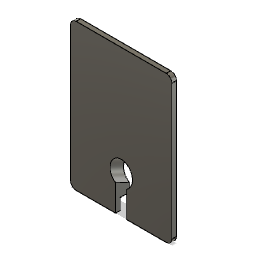
JRCNC0008 v3 (Autodesk Fusion 360 design; units mm, degrees)
Autodesk Fusion 360 part; units mm, degrees
sketch "Sketch1" plane through (0, 0, 0) normal (0, 0, 1) x (1, 0, 0)
  line L0 (0, 0) -> (114.3, 0)
  line L1 (114.3, 0) -> (114.3, 165.1)
  line L2 (114.3, 165.1) -> (0, 165.1)
  line L3 (0, 165.1) -> (0, 0)
  dimension "d19" = 114.3
  dimension "d20" = 165.1
  constraint horizontal L0
  constraint vertical L1
  constraint horizontal L2
  constraint vertical L3
  constraint coincident L0.start L3.end
  measures "d19" distance of L0.start L0.end
  measures "d20" distance of L0.start L2.end
extrude "Extrude1" add sketch "Sketch1" along normal blind 15.24
ref_plane "WorkPlane2" through (57.15, 165.1, 15.24) normal (0, 0.422618, 0.906308) x (-1, 0, 0)
sketch "Sketch2" plane through (57.15, 161.2085, 17.0546) normal (0, 0.422618, 0.906308) x (-1, 0, 0)
  circle A0 centre (0, 107.4662) radius 12.7
  line L0 (-57.15, -4.2938) -> (57.15, -4.2938) construction
  line L1 (0, -4.2938) -> (0, 107.4662)
  point P0 (57.15, -4.2938)
  point P1 (-57.15, -4.2938)
  dimension "d21" = 111.76
  dimension "d23" = 25.4
  constraint horizontal L0
  constraint coincident P0 L0.end
  constraint coincident P1 L0.start
  constraint midpoint L0 L1.start
  constraint perpendicular L0 L1
  constraint coincident A0.centre L1.end
  measures "d21" distance of L1.start A0.centre
  measures "d23" diameter of A0
extrude "Extrude2" cut sketch "Sketch2" against normal blind 203.2
sketch "Sketch3" plane through (114.3, 0, 0) normal (1, 0, 0) x (0, 1, 0)
  line L0 (0, 0) -> (165.1, 0)
  line L1 (165.1, 0) -> (165.1, 15.24)
  line L2 (165.1, 15.24) -> (0, 15.24)
  line L3 (0, 15.24) -> (0, 0)
  line L4 (133.35, 15.24) -> (88.9, 15.24)
  line L5 (88.9, 15.24) -> (88.9, 80.645)
  line L6 (88.9, 80.645) -> (133.35, 80.645)
  line L7 (133.35, 80.645) -> (133.35, 15.24)
  line L8 (133.35, 72.39) -> (107.95, 72.39)
  line L9 (107.95, 72.39) -> (107.95, 43.815)
  line L10 (107.95, 43.815) -> (133.35, 43.815)
  line L11 (133.35, 43.815) -> (133.35, 72.39)
  dimension "d22" = 28.575
  dimension "d24" = 57.15
  dimension "d25" = 25.4
  dimension "d26" = 8.255
  dimension "d27" = 19.05
  dimension "d28" = 88.9
  constraint horizontal L4
  constraint vertical L5
  constraint horizontal L6
  constraint vertical L7
  constraint coincident L2 L4.start
  constraint horizontal L8
  constraint vertical L9
  constraint horizontal L10
  constraint vertical L11
  constraint coincident L7 L8.start
  measures "d22" distance of L8.end L9.end
  measures "d24" distance of L4 L8
  measures "d25" distance of L8.start L8.end
  measures "d26" distance of L6.end L8
  measures "d27" distance of L5 L9
  measures "d28" distance of L3 L5
sketch "Sketch4" plane through (0, 0, 0) normal (0, 0, -1) x (1, 0, 0)
  line L0 (0, 0) -> (0, -165.1)
  line L1 (0, -165.1) -> (114.3, -165.1)
  line L2 (114.3, -165.1) -> (114.3, 0)
  line L3 (114.3, 0) -> (0, 0)
  line L4 (0, 0) -> (114.3, 0)
  line L5 (114.3, 0) -> (114.3, -165.1)
  line L6 (114.3, -165.1) -> (0, -165.1)
  line L7 (0, -165.1) -> (0, 0)
  line L8 (57.15, 0) -> (57.15, -165.1) construction
  line L9 (101.6, -12.7) -> (12.7, -12.7)
  line L10 (12.7, -12.7) -> (12.7, -152.4)
  line L11 (12.7, -152.4) -> (101.6, -152.4)
  line L12 (101.6, -152.4) -> (101.6, -12.7)
  line L13 (101.6, -12.7) -> (12.7, -152.4) construction
  line L14 (12.7, -12.7) -> (101.6, -152.4) construction
  line L15 (0, -82.55) -> (114.3, -82.55) construction
  ellipse E0 centre (57.15, -34.68) end of major axis (57.15, -48.6929) minor radius 12.7
  point P0 (57.15, -82.55)
  dimension "d17" = 88.9
  dimension "d18" = 139.7
  constraint horizontal L4
  constraint vertical L5
  constraint horizontal L6
  constraint vertical L7
  constraint coincident L1.end L2.start
  constraint coincident L0.start L3.end
  constraint midpoint L4 L8.start
  constraint midpoint L6 L8.end
  constraint horizontal L9
  constraint perpendicular L9 L10
  constraint parallel L9 L11
  constraint parallel L10 L12
  constraint coincident L13 P0
  constraint coincident L14 P0
  constraint coincident L8 P0
  constraint midpoint L7 L15.start
  constraint midpoint L2 L15.end
  constraint midpoint L8 P0
  measures "d17" distance of L9.start L9.end
  measures "d18" distance of L9.start L11.end
extrude "Extrude4" cut sketch "Sketch4" against normal blind 10.16 contours L0 L1 L2 L3 L4 L5 L6 L7
fillet "Fillet2" radius 6.35 8 edges at (114.3, 0, 12.7) (0, 0, 12.7) (114.3, 165.1, 12.7) (0, 165.1, 12.7) (12.7, 152.4, 5.08) (12.7, 12.7, 5.08) (101.6, 152.4, 5.08) (101.6, 12.7, 5.08)
sketch "Sketch6" plane through (0, 0, 15.24) normal (0, 0, 1) x (-1, 0, 0)
  arc A0 (-6.35, -165.1) -> (0, -158.75) centre (-6.35, -158.75) ccw
  line L0 (0, -158.75) -> (0, -6.35)
  arc A1 (0, -6.35) -> (-6.35, 0) centre (-6.35, -6.35) ccw
  line L1 (-6.35, 0) -> (-107.95, 0)
  arc A2 (-107.95, 0) -> (-114.3, -6.35) centre (-107.95, -6.35) ccw
  line L2 (-114.3, -6.35) -> (-114.3, -158.75)
  arc A3 (-114.3, -158.75) -> (-107.95, -165.1) centre (-107.95, -158.75) ccw
  line L3 (-107.95, -165.1) -> (-6.35, -165.1)
  ellipse E0 centre (-57.15, -41.7865) end of major axis (-57.15, -55.7994) minor radius 12.7
  line L4 (-57.15, -165.1) -> (-57.15, 0)
  line L5 (-50.8, 0) -> (-63.5, 0)
  line L6 (-63.5, 0) -> (-63.5, -29.651)
  line L7 (-63.5, -29.651) -> (-50.8, -29.651)
  line L8 (-50.8, -29.651) -> (-50.8, 0)
  line L9 (-50.8, 0) -> (-63.5, -29.651) construction
  line L10 (-63.5, 0) -> (-50.8, -29.651) construction
  point P0 (-57.15, -14.8255)
  dimension "d59" = 12.7
  constraint midpoint L3 L4.start
  constraint midpoint L1 L4.end
  constraint horizontal L5
  constraint perpendicular L5 L6
  constraint parallel L5 L7
  constraint parallel L6 L8
  constraint coincident L1 L5.start
  constraint coincident L9 P0
  constraint coincident L10 P0
  constraint coincident L4 P0
  constraint coincident E0 L6.end
  measures "d59" distance of L6.end L7.end
extrude "Extrude8" cut sketch "Sketch6" against normal blind 50.8 contours L1 E0 L4 L5 L8 | L1 E0 L4 L5 L6
shell "Shell2" thickness 5.08 removed faces 1 at (57.15, 113.5976, 0)
